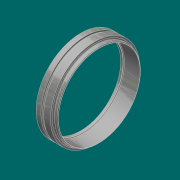
# Autodesk Inventor part: A1-19027-400-05 36in Type B Victaulic ring
Saved by Autodesk Inventor 2017.3 (Build 213256000, 256)
## iProperties
Created: 2014-07-03
Part Number: A1-19027-400-05 36in Type B Victaulic ring
Material: Steel, Mild
Document SubType Name: Modeling
Designer: Graeme_Van_Dongen
Density: 7.86 g/cm^3
Appearance: Steel
Description: 36" TYPE B VICTAULIC RING FOR STYLE 2xx COUPLING - CUSTOM, A105N
Mass: 155811 g
Surface Area: 15132.6 cm^2
Volume: 19823.3 cm^3
Author: Graeme_Van_Dongen
Autodesk Inventor part; units mm, degrees
ref_plane "YZ Plane" through (0, 0, 0) normal (1, 0, 0) x (0, 1, 0)
ref_plane "XZ Plane" through (0, 0, 0) normal (0, 1, 0) x (-1, 0, 0)
ref_plane "XY Plane" through (0, 0, 0) normal (0, 0, 1) x (1, 0, 0)
sketch "Sketch1" plane through (0, 0, 0) normal (0, 0, 1) x (1, 0, 0)
  line L0 (0, 438.15) -> (0, 488.95)
  line L1 (0, 488.95) -> (52.07, 488.95)
  line L2 (52.07, 488.95) -> (54.7572, 473.71)
  line L3 (54.7572, 473.71) -> (77.4902, 473.71)
  line L4 (77.4902, 473.71) -> (83.0371, 488.95)
  line L5 (83.0371, 488.95) -> (157.1625, 488.95)
  line L6 (157.1625, 488.95) -> (157.1625, 469.9)
  line L7 (169.8625, 457.2) -> (197.1093, 457.2)
  line L8 (197.1093, 457.2) -> (203.2, 449.2625)
  line L9 (203.2, 447.675) -> (31.75, 447.675)
  line L10 (25.4, 441.325) -> (25.4, 438.15)
  line L11 (25.4, 438.15) -> (0, 438.15)
  arc A0 (31.75, 447.675) -> (25.4, 441.325) centre (31.75, 441.325) ccw
  line L12 (-40.64, 0) -> (243.84, 0) projected
  arc A1 (157.1625, 469.9) -> (169.8625, 457.2) centre (169.8625, 469.9) ccw
  line L13 (203.2, 447.675) -> (203.2, 449.2625)
  point P0 (0, 0)
  dimension "d0" = 488.95
  dimension "d1" = 157.1625
  dimension "d3" = 457.2
  dimension "d5" = 7.9375
  dimension "d10" = 6.35
  dimension "d12" = 438.15
  dimension "d13" = 52.07
  dimension "d17" = 9.525
  dimension "d32" = 12.7
  dimension "d35" = 25.4
  dimension "d38" = 10
  dimension "d39" = 20
  dimension "d40" = 22.733
  dimension "d41" = 15.24
  dimension "d44" = 203.2
  dimension "d45" = 37.5
  dimension "d47" = 9.525
  constraints: 26 end point, 6 parallel, 4 point on circle, 4 tangent, 2 centre point, 2 collinear, 2 vertical, 1 perpendicular, 1 point on line
  measures "d0" distance from line of point (0, 0) L1
  measures "d1" distance between parallel lines of L6 L0
  measures "d3" distance from line of point (0, 0) L7
  measures "d5" vertical distance of L8.end L7.end
  measures "d10" radius of A0
  measures "d12" distance from line of point (0, 0) L11
  measures "d13" distance of L0.end L1.end
  measures "d17" distance between parallel lines of L11 L9
  measures "d32" radius of A1
  measures "d35" distance between parallel lines of L10 L0
  measures "d38" angle of L0 L2
  measures "d39" angle of L0 L4
  measures "d40" distance of L2.end L3.end
  measures "d41" distance between parallel lines of L1 L3
  measures "d44" distance between parallel lines of L13 L0
  measures "d45" angle of L13 L8
  measures "d47" distance between parallel lines of L9 L7
revolve "Revolution1" add sketch "Sketch1" angle 360 about axis through (-10, 0, 0) along (1, 0, 0)
chamfer "Chamfer2" distance 0.7937 angle 45 1 edges at (25.4, -438.15, 0)
body "Solid1"
